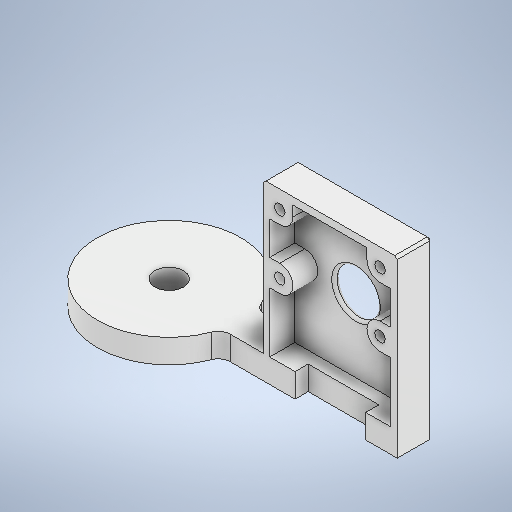
# Autodesk Inventor part: Top R
Saved by Autodesk Inventor 2025.2 (Build 292293000, 293)
## iProperties
Created: 2025-04-01
Part Number: Top R
Material: PC/ABS Plastic
Document SubType Name: Modeling
Designer: franc
Density: 1.1 g/cm^3
Appearance: Smooth - White
Author: franc
## iProperties of the stored document Top R_3DPrint.ipt
Created: 2025-04-11
Part Number: Top R_3DPrint
Material: Generic
Document SubType Name: Modeling
Designer: franc
Density: 1 g/cm^3
Appearance: Default
Author: franc
Autodesk Inventor part; units mm, degrees
ref_plane "YZ Plane" through (0, 0, 0) normal (1, 0, 0) x (0, 1, 0)
ref_plane "XZ Plane" through (0, 0, 0) normal (0, 1, 0) x (-1, 0, 0)
ref_plane "XY Plane" through (0, 0, 0) normal (0, 0, 1) x (1, 0, 0)
sketch "Sketch1" plane through (0, 0, 0) normal (0, 0, 1) x (1, 0, 0)
  line L0 (0, 0) -> (-25, 0)
  line L1 (-25, 25) -> (0, 25)
  line L2 (0, 25) -> (0, 0)
  circle A0 centre (-23.1, 22.7984) radius 1.1
  circle A1 centre (-2.1, 22.8) radius 1.1
  circle A2 centre (-23.1, 10.2984) radius 1.1
  circle A3 centre (-2.1, 10.3) radius 1.1
  line L3 (-25, 0) -> (-25.2, 0)
  line L4 (-25.2, 0) -> (-25.2, 25)
  line L5 (-25.2, 25) -> (-25, 25)
  dimension "d2" = 2.2
  dimension "d5" = 2.2
  dimension "d7" = 12.5
  dimension "d8" = 2.2
  dimension "d9" = 2.2
  dimension "d14" = 12.5
  dimension "d31" = 2.1
  dimension "d46" = 0.2
  dimension "d47" = 2.1
  dimension "d48" = 2.1
  constraints: 12 end point, 4 centre point, 2 horizontal, 2 perpendicular, 1 coincident, 1 parallel
  measures "d2" diameter of A0
  measures "d5" diameter of A1
  measures "d7" distance of point (-23.1, 10.298) A0.centre
  measures "d8" diameter of A2
  measures "d9" diameter of A3
  measures "d14" distance of A3.centre A1.centre
  measures "d31" distance from line of L2 A1.centre
  measures "d46" distance of L0.end L3.end
  measures "d47" distance from line of L4 A0.centre
  measures "d48" distance from line of L4 A2.centre
extrude "Base" add sketch "Sketch1" along normal blind 2
sketch "Sketch2" plane through (0, 0, 2) normal (0, 0, 1) x (1, 0, 0)
  line L0 (-26.5, 0) -> (-26.5, 26.5)
  line L1 (-26.5, 26.5) -> (1.5, 26.5)
  line L2 (1.5, 26.5) -> (1.5, 0)
  line L3 (1.5, 0) -> (0, 0)
  line L4 (0, 25) -> (-25.2, 25) projected
  line L5 (0, 0) -> (0, 25) projected
  line L6 (-25.2, 25) -> (-25.2, 0) projected
  line L7 (-25.2, 0) -> (-26.5, 0)
  point P0 (-25, 25)
  point P1 (-25, 0)
  dimension "d16" = 26.5
  dimension "d17" = 28
  constraints: 10 end point, 3 perpendicular, 1 horizontal
  measures "d16" distance of L0.start L0.end
  measures "d17" distance of L0.end L1.end
extrude "Walls" add sketch "Sketch2" along normal blind 5.25 and the other way blind 2
sketch "Sketch3" plane through (0, 0, 2) normal (0, 0, 1) x (1, 0, 0)
  circle A0 centre (-23.1, 10.2984) radius 1.1 projected
  circle A1 centre (-23.1, 10.2984) radius 1.6
  circle A2 centre (-2.1, 10.3) radius 1.1 projected
  circle A3 centre (-2.1, 10.3) radius 1.6
  circle A4 centre (-23.1, 22.7984) radius 1.1 projected
  circle A5 centre (-23.1, 22.7984) radius 1.6
  circle A6 centre (-2.1, 22.8) radius 1.1 projected
  circle A7 centre (-2.1, 22.8) radius 1.6
  point P0 (0, 0)
  dimension "d22" = 3.2
  dimension "d23" = 3.2
  dimension "d24" = 3.2
  dimension "d25" = 3.2
  constraints: 4 centre point, 4 coincident
  measures "d22" diameter of A1
  measures "d23" diameter of A3
  measures "d24" diameter of A5
  measures "d25" diameter of A7
extrude "Spacers" add sketch "Sketch3" along normal up to surface (5.25 mm away)
sketch "Sketch4" plane through (0, 0, 2) normal (0, 0, 1) x (1, 0, 0)
  circle A0 centre (-23.1, 10.2984) radius 1.1 projected
  arc A1 (-23.1938, 7.55) -> (-23.1, 13.0484) centre (-23.1, 10.2984) ccw
  circle A2 centre (-2.1, 10.3) radius 1.1 projected
  arc A3 (-2.1, 13.05) -> (-2.1, 7.55) centre (-2.1, 10.3) ccw
  circle A4 centre (-23.1, 22.7984) radius 1.1 projected
  circle A5 centre (-2.1, 22.8) radius 1.1 projected
  line L0 (-4.85, 22.8) -> (-4.85, 25)
  line L1 (-25.2, 25) -> (0, 25) projected
  line L2 (-2.1, 20.05) -> (0, 20.05)
  line L3 (0, 25) -> (0, 0) projected
  line L4 (-2.1, 13.05) -> (0, 13.05)
  line L5 (-2.1, 7.55) -> (0, 7.55)
  line L6 (-23.1, 13.0484) -> (-25.2, 13.0484)
  line L7 (-23.1938, 7.55) -> (-25, 7.55)
  arc A6 (-4.85, 22.8) -> (-2.1, 20.05) centre (-2.1, 22.8) ccw
  line L8 (-25, 7.55) -> (-25.2, 7.55)
  line L9 (-25.2, 13.0484) -> (-25.2, 13.0484)
  line L10 (-25.2, 25) -> (-25.2, 0) projected
  line L11 (-25.2, 20.0484) -> (-25.2, 20.0484)
  line L12 (-20.35, 22.7984) -> (-20.35, 25.6874)
  line L13 (-23.1, 20.0484) -> (-25.85, 20.0484)
  arc A7 (-23.1, 20.0484) -> (-20.35, 22.7984) centre (-23.1, 22.7984) ccw
  point P0 (-25, 25)
  point P1 (-20.35, 25)
  point P2 (-25.2, 20.0484)
  dimension "d33" = 5.5
  dimension "d34" = 5.5
  constraints: 22 end point, 8 point on circle, 7 point on line, 4 centre point, 4 coincident, 4 horizontal, 4 tangent, 3 perpendicular, 2 vertical
  measures "d33" diameter of A1
  measures "d34" diameter of A3
extrude "Spacer blocks" add sketch "Sketch4" along normal up to surface (5.25 mm away)
sketch "Sketch5" plane through (0, 0, 0) normal (0, 0, -1) x (-1, 0, 0)
  line L0 (-1.5, 26.5) -> (-1.5, 0) projected
  circle A0 centre (12.4, 10.3) radius 4.5
  point P0 (0, 0)
  dimension "d39" = 13.9
  dimension "d40" = 9
  constraints: 1 centre point, 1 coincident
  measures "d39" distance from line of point (12.4, 10.3) L0
  measures "d40" diameter of A0
extrude "Camera Hole" cut sketch "Sketch5" against normal through all
fillet "Outside Fillet - 2mm" radius 2 1 edges at (-7.9, 10.3, 0)
fillet "Inside Fillet - 1mm" radius 0.5 2 edges at (-7.9, 10.3, 1.9999) (-7.9, 10.3, 2)
chamfer "Chamfer1" distance 0.5 angle 45 5 edges at (1.5, 13.25, 0) (1.5, 26.5, 3.625) (-12.5, 26.5, 0) (-26.5, 26.5, 3.625) (-26.5, 13.25, 0)
sketch "Sketch6" plane through (-25.2, 0, 2) normal (0, -1, 0) x (1, 0, 0)
  line L0 (-0.8, -2) -> (-1.3, -1.5) projected
  line L1 (26.2, -2) -> (-0.8, -2) projected
  line L2 (26.7, -1.5) -> (26.2, -2) projected
  line L3 (26.7, -1.5) -> (26.7, 5.25) projected
  line L4 (25.2, 5.25) -> (26.7, 5.25) projected
  line L5 (25.2, 0) -> (25.2, 5.25) projected
  line L6 (0, 0) -> (25.2, 0) projected
  line L7 (0, 0) -> (0, 5.25) projected
  line L8 (-1.3, 5.25) -> (0, 5.25) projected
  line L9 (-1.3, -1.5) -> (-1.3, 5.25) projected
  point P0 (25.2, -2)
extrude "Bottom Extension" add sketch "Sketch6" along normal blind 5
sketch "Sketch7" plane through (-25.2, -5, 2) normal (0, -1, 0) x (1, 0, 0)
  line L0 (26.7, 5.25) -> (25.2, 5.25) projected
  line L1 (26.7, 5.25) -> (20.1, 5.25)
  line L2 (20.1, 5.25) -> (20.1, -2)
  line L3 (26.7, 5.25) -> (25.2, 5.25) construction
  line L4 (25.2, 5.25) -> (25.2, 0) construction
  line L5 (25.2, 0) -> (0, 0) construction
  line L6 (0, 0) -> (0, 5.25) construction
  line L7 (0, 5.25) -> (-1.3, 5.25) construction
  line L8 (-1.3, 5.25) -> (-1.3, -1.5) construction
  line L9 (-1.3, -1.5) -> (-0.8, -2) construction
  line L10 (-0.8, -2) -> (26.2, -2) construction
  line L11 (26.2, -2) -> (26.7, -1.5) construction
  line L12 (26.7, -1.5) -> (26.7, 5.25) construction
  line L13 (20.1, -2) -> (-0.8, -2)
  line L14 (-1.3, -1.5) -> (-0.8, -2)
  line L15 (-1.3, -1.5) -> (-1.3, 5.25)
  line L16 (-1.3, 5.25) -> (0, 5.25)
  line L17 (0, 5.25) -> (5.3, 5.25)
  line L18 (5.3, 5.25) -> (5.3, 0)
  line L19 (5.3, 0) -> (20.1, 0)
  line L20 (5.3, 0) -> (5.3, 2.5)
  line L21 (5.3, 2.5) -> (20.1, 2.5)
  line L22 (26.7, 5.25) -> (26.7, -1.5)
  line L23 (26.2, -2) -> (26.7, -1.5)
  line L24 (20.1, -2) -> (26.2, -2)
  line L25 (5.3, 5.25) -> (-24.7, 5.25)
  line L26 (-24.7, 5.25) -> (-24.7, -2)
  line L27 (-24.7, -2) -> (-0.8, -2)
  point P0 (25.2, -2)
  point P1 (50.1, 5.25)
  dimension "d54" = 6.6
  dimension "d58" = 5.3
  dimension "d59" = 2.5
  dimension "d68" = 30
  constraints: 34 end point, 8 point on line, 7 perpendicular, 5 collinear, 1 horizontal
  measures "d54" distance of L0.start L1.end
  measures "d58" distance of L6.end L17.end
  measures "d59" distance of L18.end L20.end
  measures "d68" distance of L17.end L25.end
extrude "Mounting Arm" add sketch "Sketch7" along normal blind 5
sketch "Sketch10" plane through (-25.2, -5, 2) normal (0, 1, 0) x (1, 0, 0)
  line L0 (-24.7, -5.25) -> (-24.7, 2) projected
  circle A0 centre (-24.7, -1.625) radius 15
  point P0 (25.2, 2)
  dimension "d69" = 30
  constraints: 1 centre point, 1 midpoint
  measures "d69" diameter of A0
extrude "Extrusion10" add sketch "Sketch10" against normal blind 5
sketch "Sketch11" plane through (-25.2, -5, 2) normal (0, 1, 0) x (1, 0, 0)
  arc A0 (-10.1446, 2) -> (-10.1446, -5.25) centre (-24.7, -1.625) ccw projected
  circle A1 centre (-24.7, -1.625) radius 3
  point P0 (25.2, 2)
  dimension "d72" = 6
  constraints: 1 centre point, 1 coincident
  measures "d72" diameter of A1
extrude "Extrusion11" cut sketch "Sketch11" against normal through all
fillet "Fillet6" radius 2.5 2 edges at (-35.3446, -7.5, 7.25) (-35.3446, -7.5, 0)
body "Solid1"
